Autodesk Inventor part; units mm, degrees
(part 3 of 7)
  line L1708 (-161.6517, 7.6453) -> (-161.371, 7.5772)
  line L1709 (-161.371, 7.5772) -> (-161.0973, 7.4847)
  line L1710 (-161.0973, 7.4847) -> (-160.8323, 7.3684)
  line L1711 (-160.8323, 7.3684) -> (-160.4964, 7.1575)
  line L1712 (-160.4964, 7.1575) -> (-160.1956, 6.9075)
  line L1713 (-160.1956, 6.9075) -> (-159.9378, 6.6106)
  line L1714 (-159.9378, 6.6106) -> (-159.719, 6.2747)
  line L1715 (-159.719, 6.2747) -> (-159.5477, 5.9087)
  line L1716 (-159.5477, 5.9087) -> (-159.4222, 5.5247)
  line L1717 (-159.4222, 5.5247) -> (-159.3479, 5.1262)
  line L1718 (-159.3479, 5.1262) -> (-159.3206, 4.7083)
  line L1719 (-159.3206, 4.7083) -> (-159.3319, 4.394)
  line L1720 (-159.3319, 4.394) -> (-159.3724, 4.0828)
  line L1721 (-159.3724, 4.0828) -> (-159.4417, 3.7767)
  line L1722 (-159.4417, 3.7767) -> (-159.5394, 3.4778)
  line L1723 (-159.5394, 3.4778) -> (-159.6691, 3.2001)
  line L1724 (-159.6691, 3.2001) -> (-159.8274, 2.9409)
  line L1725 (-159.8274, 2.9409) -> (-160.0121, 2.7021)
  line L1726 (-160.0121, 2.7021) -> (-160.2213, 2.4856)
  line L1727 (-160.2213, 2.4856) -> (-160.453, 2.2932)
  line L1728 (-160.453, 2.2932) -> (-160.705, 2.127)
  line L1729 (-160.705, 2.127) -> (-160.9754, 1.9886)
  line L1730 (-160.9754, 1.9886) -> (-161.262, 1.8801)
  line L1731 (-161.262, 1.8801) -> (-161.7812, 1.7492)
  line L1732 (-161.7812, 1.7492) -> (-162.3128, 1.6848)
  line L1733 (-162.3128, 1.6848) -> (-162.7199, 1.6679)
  line L1734 (-162.7199, 1.6679) -> (-163.1263, 1.6832)
  line L1735 (-163.1263, 1.6832) -> (-163.5304, 1.7305)
  line L1736 (-163.5304, 1.7305) -> (-163.93, 1.8098)
  line L1737 (-163.93, 1.8098) -> (-164.1821, 1.8844)
  line L1738 (-164.1821, 1.8844) -> (-164.4265, 1.9799)
  line L1739 (-164.4265, 1.9799) -> (-164.6619, 2.0959)
  line L1740 (-164.6619, 2.0959) -> (-164.887, 2.2317)
  line L1741 (-164.887, 2.2317) -> (-165.1134, 2.4105)
  line L1742 (-165.1134, 2.4105) -> (-165.3189, 2.6097)
  line L1743 (-165.3189, 2.6097) -> (-165.5025, 2.8275)
  line L1744 (-165.5025, 2.8275) -> (-165.6629, 3.062)
  line L1745 (-165.6629, 3.062) -> (-165.7992, 3.3114)
  line L1746 (-165.7992, 3.3114) -> (-165.91, 3.5738)
  line L1747 (-165.91, 3.5738) -> (-165.9944, 3.8473)
  line L1748 (-165.9944, 3.8473) -> (-166.0511, 4.1301)
  line L1749 (-166.0511, 4.1301) -> (-166.0959, 4.5823)
  line L1750 (-166.0959, 4.5823) -> (-166.0823, 5.0364)
  line L1751 (-162.1487, -31.7214) -> (-161.6707, -31.7085)
  line L1752 (-161.6707, -31.7085) -> (-161.1956, -31.655)
  line L1753 (-161.1956, -31.655) -> (-160.9008, -31.547)
  line L1754 (-160.9008, -31.547) -> (-160.6503, -31.367)
  line L1755 (-160.6503, -31.367) -> (-160.4566, -31.1269)
  line L1756 (-160.4566, -31.1269) -> (-160.3323, -30.8386)
  line L1757 (-160.3323, -30.8386) -> (-160.2843, -30.6013)
  line L1758 (-160.2843, -30.6013) -> (-160.2692, -30.363)
  line L1759 (-160.2692, -30.363) -> (-160.2861, -30.1269)
  line L1760 (-160.2861, -30.1269) -> (-160.3342, -29.896)
  line L1761 (-160.3342, -29.896) -> (-160.4126, -29.6737)
  line L1762 (-160.4126, -29.6737) -> (-160.5203, -29.4629)
  line L1763 (-160.5203, -29.4629) -> (-160.6566, -29.2668)
  line L1764 (-160.6566, -29.2668) -> (-160.8206, -29.0886)
  line L1765 (-160.8206, -29.0886) -> (-161.0047, -28.9477)
  line L1766 (-161.0047, -28.9477) -> (-161.2112, -28.8425)
  line L1767 (-161.2112, -28.8425) -> (-161.6426, -28.7268)
  line L1768 (-161.6426, -28.7268) -> (-162.0862, -28.6746)
  line L1769 (-162.0862, -28.6746) -> (-162.4769, -28.6628)
  line L1770 (-162.4769, -28.6628) -> (-165.9495, -28.6628)
  line L1771 (-165.9495, -28.6628) -> (-165.9495, -27.5652)
  line L1772 (-165.9495, -27.5652) -> (-159.469, -27.5652)
  line L1773 (-159.469, -27.5652) -> (-159.469, -28.5496)
  line L1774 (-159.469, -28.5496) -> (-160.4222, -28.5496)
  line L1775 (-160.4222, -28.5496) -> (-160.234, -28.6876)
  line L1776 (-160.234, -28.6876) -> (-160.0587, -28.841)
  line L1777 (-160.0587, -28.841) -> (-159.8971, -29.0088)
  line L1778 (-159.8971, -29.0088) -> (-159.7503, -29.1902)
  line L1779 (-159.7503, -29.1902) -> (-159.5954, -29.4431)
  line L1780 (-159.5954, -29.4431) -> (-159.4745, -29.7126)
  line L1781 (-159.4745, -29.7126) -> (-159.389, -29.9953)
  line L1782 (-159.389, -29.9953) -> (-159.3401, -30.2878)
  line L1783 (-159.3401, -30.2878) -> (-159.3229, -30.7084)
  line L1784 (-159.3229, -30.7084) -> (-159.3716, -31.1238)
  line L1785 (-159.3716, -31.1238) -> (-159.4846, -31.5266)
  line L1786 (-159.4846, -31.5266) -> (-159.6604, -31.9089)
  line L1787 (-159.6604, -31.9089) -> (-159.812, -32.1381)
  line L1788 (-159.812, -32.1381) -> (-159.9997, -32.3358)
  line L1789 (-159.9997, -32.3358) -> (-160.219, -32.4978)
  line L1790 (-160.219, -32.4978) -> (-160.4651, -32.6199)
  line L1791 (-160.4651, -32.6199) -> (-160.7422, -32.7101)
  line L1792 (-160.7422, -32.7101) -> (-161.026, -32.7729)
  line L1793 (-161.026, -32.7729) -> (-161.3145, -32.8081)
  line L1794 (-161.3145, -32.8081) -> (-161.6058, -32.8152)
  line L1795 (-161.6058, -32.8152) -> (-161.9339, -32.8191)
  line L1796 (-161.9339, -32.8191) -> (-165.9495, -32.8191)
  line L1797 (-165.9495, -32.8191) -> (-165.9495, -31.7214)
  line L1798 (-165.9495, -31.7214) -> (-162.1487, -31.7214)
  line L1799 (-166.0823, 18.9309) -> (-166.0294, 19.3048)
  line L1800 (-166.0294, 19.3048) -> (-165.9272, 19.6627)
  line L1801 (-165.9272, 19.6627) -> (-165.7786, 20.0006)
  line L1802 (-165.7786, 20.0006) -> (-165.5867, 20.314)
  line L1803 (-165.5867, 20.314) -> (-165.3544, 20.5989)
  line L1804 (-165.3544, 20.5989) -> (-165.0848, 20.8509)
  line L1805 (-165.0848, 20.8509) -> (-164.7809, 21.0658)
  line L1806 (-164.7809, 21.0658) -> (-164.4456, 21.2395)
  line L1807 (-164.4456, 21.2395) -> (-164.1239, 21.3614)
  line L1808 (-164.1239, 21.3614) -> (-163.7934, 21.4544)
  line L1809 (-163.7934, 21.4544) -> (-163.4559, 21.5181)
  line L1810 (-163.4559, 21.5181) -> (-163.1136, 21.552)
  line L1811 (-163.1136, 21.552) -> (-162.7718, 21.561)
  line L1812 (-162.7718, 21.561) -> (-162.43, 21.5559)
  line L1813 (-162.43, 21.5559) -> (-162.43, 16.7239)
  line L1814 (-162.43, 16.7239) -> (-162.1358, 16.7468)
  line L1815 (-162.1358, 16.7468) -> (-161.8463, 16.7991)
  line L1816 (-161.8463, 16.7991) -> (-161.5634, 16.8801)
  line L1817 (-161.5634, 16.8801) -> (-161.2894, 16.9895)
  line L1818 (-161.2894, 16.9895) -> (-161.0538, 17.1191)
  line L1819 (-161.0538, 17.1191) -> (-160.8431, 17.2792)
  line L1820 (-160.8431, 17.2792) -> (-160.6596, 17.4661)
  line L1821 (-160.6596, 17.4661) -> (-160.5054, 17.6765)
  line L1822 (-160.5054, 17.6765) -> (-160.3829, 17.9067)
  line L1823 (-160.3829, 17.9067) -> (-160.2941, 18.1532)
  line L1824 (-160.2941, 18.1532) -> (-160.2413, 18.4124)
  line L1825 (-160.2413, 18.4124) -> (-160.2269, 18.6809)
  line L1826 (-160.2269, 18.6809) -> (-160.2451, 18.965)
  line L1827 (-160.2451, 18.965) -> (-160.305, 19.2434)
  line L1828 (-160.305, 19.2434) -> (-160.4023, 19.4889)
  line L1829 (-160.4023, 19.4889) -> (-160.5433, 19.7122)
  line L1830 (-160.5433, 19.7122) -> (-160.7325, 19.9205)
  line L1831 (-160.7325, 19.9205) -> (-160.9534, 20.095)
  line L1832 (-160.9534, 20.095) -> (-161.2449, 20.2622)
  line L1833 (-161.2449, 20.2622) -> (-161.555, 20.3918)
  line L1834 (-161.555, 20.3918) -> (-161.4144, 21.5286)
  line L1835 (-161.4144, 21.5286) -> (-161.0762, 21.42)
  line L1836 (-161.0762, 21.42) -> (-160.7548, 21.2719)
  line L1837 (-160.7548, 21.2719) -> (-160.4536, 21.0861)
  line L1838 (-160.4536, 21.0861) -> (-160.1761, 20.8645)
  line L1839 (-160.1761, 20.8645) -> (-159.9008, 20.5641)
  line L1840 (-159.9008, 20.5641) -> (-159.6771, 20.2266)
  line L1841 (-159.6771, 20.2266) -> (-159.5085, 19.8584)
  line L1842 (-159.5085, 19.8584) -> (-159.3987, 19.4661)
  line L1843 (-159.3987, 19.4661) -> (-159.3276, 18.9457)
  line L1844 (-159.3276, 18.9457) -> (-159.3283, 18.4229)
  line L1845 (-159.3283, 18.4229) -> (-159.4004, 17.9051)
  line L1846 (-159.4004, 17.9051) -> (-159.5433, 17.3997)
  line L1847 (-159.5433, 17.3997) -> (-159.6699, 17.1215)
  line L1848 (-159.6699, 17.1215) -> (-159.8254, 16.8617)
  line L1849 (-159.8254, 16.8617) -> (-160.0078, 16.6223)
  line L1850 (-160.0078, 16.6223) -> (-160.215, 16.4051)
  line L1851 (-160.215, 16.4051) -> (-160.4449, 16.2122)
  line L1852 (-160.4449, 16.2122) -> (-160.6955, 16.0454)
  line L1853 (-160.6955, 16.0454) -> (-160.9646, 15.9067)
  line L1854 (-160.9646, 15.9067) -> (-161.2503, 15.7981)
  line L1855 (-161.2503, 15.7981) -> (-161.5947, 15.7031)
  line L1856 (-161.5947, 15.7031) -> (-161.9449, 15.6361)
  line L1857 (-161.9449, 15.6361) -> (-162.2995, 15.5974)
  line L1858 (-162.2995, 15.5974) -> (-162.6565, 15.5872)
  line L1859 (-162.6565, 15.5872) -> (-163.0242, 15.5978)
  line L1860 (-163.0242, 15.5978) -> (-163.3893, 15.6367)
  line L1861 (-163.3893, 15.6367) -> (-163.7504, 15.7035)
  line L1862 (-163.7504, 15.7035) -> (-164.1058, 15.7981)
  line L1863 (-164.1058, 15.7981) -> (-164.3965, 15.9063)
  line L1864 (-164.3965, 15.9063) -> (-164.6712, 16.0443)
  line L1865 (-164.6712, 16.0443) -> (-164.9279, 16.2102)
  line L1866 (-164.9279, 16.2102) -> (-165.1647, 16.4023)
  line L1867 (-165.1647, 16.4023) -> (-165.3794, 16.6187)
  line L1868 (-165.3794, 16.6187) -> (-165.5701, 16.8576)
  line L1869 (-165.5701, 16.8576) -> (-165.7348, 17.1173)
  line L1870 (-165.7348, 17.1173) -> (-165.8714, 17.3958)
  line L1871 (-165.8714, 17.3958) -> (-165.9915, 17.7683)
  line L1872 (-165.9915, 17.7683) -> (-166.0671, 18.1509)
  line L1873 (-166.0671, 18.1509) -> (-166.0976, 18.5398)
  line L1874 (-166.0976, 18.5398) -> (-166.0823, 18.9309)
  line L1875 (-166.0862, -17.1589) -> (-166.0498, -16.8212)
  line L1876 (-166.0498, -16.8212) -> (-165.9886, -16.4871)
  line L1877 (-165.9886, -16.4871) -> (-165.9182, -16.2439)
  line L1878 (-165.9182, -16.2439) -> (-165.8211, -16.011)
  line L1879 (-165.8211, -16.011) -> (-165.6984, -15.7906)
  line L1880 (-165.6984, -15.7906) -> (-165.5511, -15.5847)
  line L1881 (-165.5511, -15.5847) -> (-165.4065, -15.444)
  line L1882 (-165.4065, -15.444) -> (-165.2447, -15.3251)
  line L1883 (-165.2447, -15.3251) -> (-165.0681, -15.2296)
  line L1884 (-165.0681, -15.2296) -> (-164.8792, -15.1589)
  line L1885 (-164.8792, -15.1589) -> (-164.5781, -15.0877)
  line L1886 (-164.5781, -15.0877) -> (-164.2698, -15.0613)
  line L1887 (-164.2698, -15.0613) -> (-163.9594, -15.0488)
  line L1888 (-163.9594, -15.0488) -> (-163.6487, -15.0457)
  line L1889 (-163.6487, -15.0457) -> (-162.4222, -15.0489)
  line L1890 (-162.4222, -15.0489) -> (-161.1956, -15.0378)
  line L1891 (-161.1956, -15.0378) -> (-160.72, -15.0223)
  line L1892 (-160.72, -15.0223) -> (-160.2464, -14.9753)
  line L1893 (-160.2464, -14.9753) -> (-160.0431, -14.933)
  line L1894 (-160.0431, -14.933) -> (-159.845, -14.8724)
  line L1895 (-159.845, -14.8724) -> (-159.6532, -14.7939)
  line L1896 (-159.6532, -14.7939) -> (-159.469, -14.698)
  line L1897 (-159.469, -14.698) -> (-159.469, -15.8464)
  line L1898 (-159.469, -15.8464) -> (-159.6611, -15.9284)
  line L1899 (-159.6611, -15.9284) -> (-159.8595, -15.9923)
  line L1900 (-159.8595, -15.9923) -> (-160.0628, -16.0381)
  line L1901 (-160.0628, -16.0381) -> (-160.2698, -16.0652)
  line L1902 (-160.2698, -16.0652) -> (-159.9385, -16.4923)
  line L1903 (-159.9385, -16.4923) -> (-159.6604, -16.9558)
  line L1904 (-159.6604, -16.9558) -> (-159.5367, -17.2459)
  line L1905 (-159.5367, -17.2459) -> (-159.4406, -17.5441)
  line L1906 (-159.4406, -17.5441) -> (-159.3723, -17.8486)
  line L1907 (-159.3723, -17.8486) -> (-159.332, -18.1574)
  line L1908 (-159.332, -18.1574) -> (-159.3198, -18.4686)
  line L1909 (-159.3198, -18.4686) -> (-159.3358, -18.7803)
  line L1910 (-159.3358, -18.7803) -> (-159.3803, -19.0905)
  line L1911 (-159.3803, -19.0905) -> (-159.4534, -19.3972)
  line L1912 (-159.4534, -19.3972) -> (-159.5274, -19.6029)
  line L1913 (-159.5274, -19.6029) -> (-159.6248, -19.7959)
  line L1914 (-159.6248, -19.7959) -> (-159.7441, -19.9743)
  line L1915 (-159.7441, -19.9743) -> (-159.8836, -20.1365)
  line L1916 (-159.8836, -20.1365) -> (-160.0415, -20.2808)
  line L1917 (-160.0415, -20.2808) -> (-160.2163, -20.4054)
  line L1918 (-160.2163, -20.4054) -> (-160.4063, -20.5085)
  line L1919 (-160.4063, -20.5085) -> (-160.6097, -20.5886)
  line L1920 (-160.6097, -20.5886) -> (-160.9739, -20.6615)
  line L1921 (-160.9739, -20.6615) -> (-161.3419, -20.6623)
  line L1922 (-161.3419, -20.6623) -> (-161.7032, -20.5921)
  line L1923 (-161.7032, -20.5921) -> (-162.0472, -20.4519)
  line L1924 (-162.0472, -20.4519) -> (-162.3151, -20.2729)
  line L1925 (-162.3151, -20.2729) -> (-162.5475, -20.0529)
  line L1926 (-162.5475, -20.0529) -> (-162.7397, -19.7971)
  line L1927 (-162.7397, -19.7971) -> (-162.887, -19.5105)
  line L1928 (-162.887, -19.5105) -> (-162.9874, -19.2476)
  line L1929 (-162.9874, -19.2476) -> (-163.0672, -18.9781)
  line L1930 (-163.0672, -18.9781) -> (-163.1263, -18.7034)
  line L1931 (-163.1263, -18.7034) -> (-163.1644, -18.4246)
  line L1932 (-163.1644, -18.4246) -> (-163.291, -17.4646)
  line L1933 (-163.291, -17.4646) -> (-163.4769, -16.5144)
  line L1934 (-163.4769, -16.5144) -> (-163.5251, -16.3354)
  line L1935 (-163.5251, -16.3354) -> (-163.5823, -16.1589)
  line L1936 (-163.5823, -16.1589) -> (-164.015, -16.158)
  line L1937 (-164.015, -16.158) -> (-164.4417, -16.2293)
  line L1938 (-164.4417, -16.2293) -> (-164.6111, -16.301)
  line L1939 (-164.6111, -16.301) -> (-164.7599, -16.4058)
  line L1940 (-164.7599, -16.4058) -> (-164.8834, -16.5395)
  line L1941 (-164.8834, -16.5395) -> (-164.9769, -16.698)
  line L1942 (-164.9769, -16.698) -> (-165.0615, -16.8928)
  line L1943 (-165.0615, -16.8928) -> (-165.1246, -17.095)
  line L1944 (-165.1246, -17.095) -> (-165.1655, -17.3028)
  line L1945 (-165.1655, -17.3028) -> (-165.1839, -17.5144)
  line L1946 (-165.1839, -17.5144) -> (-165.1827, -17.9541)
  line L1947 (-165.1827, -17.9541) -> (-165.1214, -18.3894)
  line L1948 (-165.1214, -18.3894) -> (-165.0354, -18.6472)
  line L1949 (-165.0354, -18.6472) -> (-164.9183, -18.8582)
  line L1950 (-164.9183, -18.8582) -> (-164.7542, -19.03)
  line L1951 (-164.7542, -19.03) -> (-164.5394, -19.1785)
  line L1952 (-164.5394, -19.1785) -> (-164.2539, -19.3112)
  line L1953 (-164.2539, -19.3112) -> (-163.9534, -19.405)
  line L1954 (-163.9534, -19.405) -> (-164.1019, -20.4793)
  line L1955 (-164.1019, -20.4793) -> (-164.3331, -20.4248)
  line L1956 (-164.3331, -20.4248) -> (-164.5587, -20.3517)
  line L1957 (-164.5587, -20.3517) -> (-164.7776, -20.2603)
  line L1958 (-164.7776, -20.2603) -> (-164.9886, -20.1511)
  line L1959 (-164.9886, -20.1511) -> (-165.1636, -20.0373)
  line L1960 (-165.1636, -20.0373) -> (-165.3233, -19.9039)
  line L1961 (-165.3233, -19.9039) -> (-165.466, -19.7526)
  line L1962 (-165.466, -19.7526) -> (-165.5901, -19.5847)
  line L1963 (-165.5901, -19.5847) -> (-165.7484, -19.3151)
  line L1964 (-165.7484, -19.3151) -> (-165.8675, -19.0261)
  line L1965 (-165.8675, -19.0261) -> (-166.0114, -18.5003)
  line L1966 (-166.0114, -18.5003) -> (-166.0823, -17.9597)
  line L1967 (-166.0823, -17.9597) -> (-166.0979, -17.5594)
  line L1968 (-166.0979, -17.5594) -> (-166.0862, -17.1589)
  line L1969 (-165.9495, -0.1277) -> (-165.9495, 0.9778)
  line L1970 (-165.9495, 0.9778) -> (-165.0979, 0.9778)
  line L1971 (-165.0979, 0.9778) -> (-165.0979, -0.1277)
  line L1972 (-165.0979, -0.1277) -> (-161.305, -0.1277)
  line L1973 (-161.305, -0.1277) -> (-161.0019, -0.1218)
  line L1974 (-161.0019, -0.1218) -> (-160.7034, -0.0691)
  line L1975 (-160.7034, -0.0691) -> (-160.5823, 0.009)
  line L1976 (-160.5823, 0.009) -> (-160.4886, 0.1184)
  line L1977 (-160.4886, 0.1184) -> (-160.4244, 0.3027)
  line L1978 (-160.4244, 0.3027) -> (-160.4104, 0.4973)
  line L1979 (-160.4104, 0.4973) -> (-160.4208, 0.7385)
  line L1980 (-160.4208, 0.7385) -> (-160.4534, 0.9778)
  line L1981 (-160.4534, 0.9778) -> (-159.4808, 1.1379)
  line L1982 (-159.4808, 1.1379) -> (-159.4181, 0.8002)
  line L1983 (-159.4181, 0.8002) -> (-159.3887, 0.4588)
  line L1984 (-159.3887, 0.4588) -> (-159.3926, 0.1161)
  line L1985 (-159.3926, 0.1161) -> (-159.43, -0.2253)
  line L1986 (-159.43, -0.2253) -> (-159.4939, -0.454)
  line L1987 (-159.4939, -0.454) -> (-159.5996, -0.6641)
  line L1988 (-159.5996, -0.6641) -> (-159.7435, -0.8502)
  line L1989 (-159.7435, -0.8502) -> (-159.9222, -1.0066)
  line L1990 (-159.9222, -1.0066) -> (-160.0697, -1.0786)
  line L1991 (-160.0697, -1.0786) -> (-160.2242, -1.1329)
  line L1992 (-160.2242, -1.1329) -> (-160.3838, -1.1689)
  line L1993 (-160.3838, -1.1689) -> (-160.5472, -1.1863)
  line L1994 (-160.5472, -1.1863) -> (-160.8379, -1.2064)
  line L1995 (-160.8379, -1.2064) -> (-161.1292, -1.2175)
  line L1996 (-161.1292, -1.2175) -> (-165.0979, -1.2175)
  line L1997 (-165.0979, -1.2175) -> (-165.0979, -2.0261)
  line L1998 (-165.0979, -2.0261) -> (-165.9495, -2.0261)
  line L1999 (-165.9495, -2.0261) -> (-165.9495, -1.2175)
  line L2000 (-165.9495, -1.2175) -> (-167.555, -1.2175)
  line L2001 (-167.555, -1.2175) -> (-168.2151, -0.1277)
  line L2002 (-168.2151, -0.1277) -> (-165.9495, -0.1277)
  line L2003 (-166.0745, 25.6145) -> (-166.0237, 25.8381)
  line L2004 (-166.0237, 25.8381) -> (-165.951, 26.055)
  line L2005 (-165.951, 26.055) -> (-165.857, 26.2635)
  line L2006 (-165.857, 26.2635) -> (-165.7425, 26.4621)
  line L2007 (-165.7425, 26.4621) -> (-164.7229, 26.0871)
  line L2008 (-164.7229, 26.0871) -> (-164.8424, 25.8584)
  line L2009 (-164.8424, 25.8584) -> (-164.9209, 25.6144)
  line L2010 (-164.9209, 25.6144) -> (-164.957, 25.3607)
  line L2011 (-164.957, 25.3607) -> (-164.9495, 25.1028)
  line L2012 (-164.9495, 25.1028) -> (-164.8482, 24.8038)
  line L2013 (-164.8482, 24.8038) -> (-164.6722, 24.5488)
  line L2014 (-164.6722, 24.5488) -> (-164.4337, 24.3511)
  line L2015 (-164.4337, 24.3511) -> (-164.1448, 24.2239)
  line L2016 (-164.1448, 24.2239) -> (-163.8304, 24.1419)
  line L2017 (-163.8304, 24.1419) -> (-163.5111, 24.0838)
  line L2018 (-163.5111, 24.0838) -> (-163.1884, 24.0499)
  line L2019 (-163.1884, 24.0499) -> (-162.8636, 24.0403)
  line L2020 (-162.8636, 24.0403) -> (-159.469, 24.0403)
  line L2021 (-159.469, 24.0403) -> (-159.469, 22.9426)
  line L2022 (-159.469, 22.9426) -> (-165.9495, 22.9426)
  line L2023 (-165.9495, 22.9426) -> (-165.9495, 23.9309)
  line L2024 (-165.9495, 23.9309) -> (-164.969, 23.9309)
  line L2025 (-164.969, 23.9309) -> (-165.3729, 24.171)
  line L2026 (-165.3729, 24.171) -> (-165.7386, 24.4661)
  line L2027 (-165.7386, 24.4661) -> (-165.8926, 24.6524)
  line L2028 (-165.8926, 24.6524) -> (-166.0057, 24.8634)
  line L2029 (-166.0057, 24.8634) -> (-166.0751, 25.0926)
  line L2030 (-166.0751, 25.0926) -> (-166.0979, 25.3332)
  line L2031 (-166.0979, 25.3332) -> (-166.0745, 25.6145)
  line L2032 (-159.469, -21.9402) -> (-159.469, -23.0418)
  line L2033 (-159.469, -23.0418) -> (-165.9495, -23.0418)
  line L2034 (-165.9495, -23.0418) -> (-165.9495, -21.9402)
  line L2035 (-165.9495, -21.9402) -> (-159.469, -21.9402)
  line L2036 (-159.469, -24.7214) -> (-159.469, -25.8191)
  line L2037 (-159.469, -25.8191) -> (-168.4183, -25.8191)
  line L2038 (-168.4183, -25.8191) -> (-168.4183, -24.7214)
  line L2039 (-168.4183, -24.7214) -> (-159.469, -24.7214)
  line L2040 (-162.6604, -16.3152) -> (-162.4486, -17.1258)
  line L2041 (-162.4486, -17.1258) -> (-162.3089, -17.9519)
  line L2042 (-162.3089, -17.9519) -> (-162.2265, -18.4372)
  line L2043 (-162.2265, -18.4372) -> (-162.0862, -18.9089)
  line L2044 (-162.0862, -18.9089) -> (-161.9426, -19.1525)
  line L2045 (-161.9426, -19.1525) -> (-161.7377, -19.3384)
  line L2046 (-161.7377, -19.3384) -> (-161.4873, -19.456)
  line L2047 (-161.4873, -19.456) -> (-161.2073, -19.4949)
  line L2048 (-161.2073, -19.4949) -> (-161.0015, -19.4764)
  line L2049 (-161.0015, -19.4764) -> (-160.805, -19.4128)
  line L2050 (-160.805, -19.4128) -> (-160.6666, -19.3319)
  line L2051 (-160.6666, -19.3319) -> (-160.5429, -19.2314)
  line L2052 (-160.5429, -19.2314) -> (-160.436, -19.1132)
  line L2053 (-160.436, -19.1132) -> (-160.3479, -18.9793)
  line L2054 (-160.3479, -18.9793) -> (-160.2545, -18.741)
  line L2055 (-160.2545, -18.741) -> (-160.1995, -18.491)
  line L2056 (-160.1995, -18.491) -> (-160.1809, -18.1923)
  line L2057 (-160.1809, -18.1923) -> (-160.1984, -17.8945)
  line L2058 (-160.1984, -17.8945) -> (-160.2516, -17.6011)
  line L2059 (-160.2516, -17.6011) -> (-160.3401, -17.3152)
  line L2060 (-160.3401, -17.3152) -> (-160.4251, -17.1273)
  line L2061 (-160.4251, -17.1273) -> (-160.5289, -16.9499)
  line L2062 (-160.5289, -16.9499) -> (-160.6507, -16.7841)
  line L2063 (-160.6507, -16.7841) -> (-160.7894, -16.6316)
  line L2064 (-160.7894, -16.6316) -> (-160.9931, -16.4671)
  line L2065 (-160.9931, -16.4671) -> (-161.219, -16.3347)
  line L2066 (-161.219, -16.3347) -> (-161.5906, -16.2186)
  line L2067 (-161.5906, -16.2186) -> (-161.9769, -16.1707)
  line L2068 (-161.9769, -16.1707) -> (-162.3498, -16.1584)
  line L2069 (-162.3498, -16.1584) -> (-162.7229, -16.1589)
  line L2070 (-162.7229, -16.1589) -> (-162.6604, -16.3152)
  line L2071 (-165.18, 4.509) -> (-165.1362, 4.2596)
  line L2072 (-165.1362, 4.2596) -> (-165.0591, 4.0222)
  line L2073 (-165.0591, 4.0222) -> (-164.9508, 3.7998)
  line L2074 (-164.9508, 3.7998) -> (-164.8136, 3.5953)
  line L2075 (-164.8136, 3.5953) -> (-164.6496, 3.4115)
  line L2076 (-164.6496, 3.4115) -> (-164.4612, 3.2512)
  line L2077 (-164.4612, 3.2512) -> (-164.2505, 3.1174)
  line L2078 (-164.2505, 3.1174) -> (-164.0198, 3.0129)
  line L2079 (-164.0198, 3.0129) -> (-163.7012, 2.9138)
  line L2080 (-163.7012, 2.9138) -> (-163.3755, 2.8448)
  line L2081 (-163.3755, 2.8448) -> (-163.0448, 2.8061)
  line L2082 (-163.0448, 2.8061) -> (-162.7112, 2.7981)
  line L2083 (-162.7112, 2.7981) -> (-162.4357, 2.8037)
  line L2084 (-162.4357, 2.8037) -> (-162.1615, 2.8284)
  line L2085 (-162.1615, 2.8284) -> (-161.8898, 2.8722)
  line L2086 (-161.8898, 2.8722) -> (-161.6214, 2.9348)
  line L2087 (-161.6214, 2.9348) -> (-161.4121, 3.0059)
  line L2088 (-161.4121, 3.0059) -> (-161.2118, 3.0979)
  line L2089 (-161.2118, 3.0979) -> (-161.0219, 3.2099)
  line L2090 (-161.0219, 3.2099) -> (-160.844, 3.3411)
  line L2091 (-160.844, 3.3411) -> (-160.685, 3.4959)
  line L2092 (-160.685, 3.4959) -> (-160.5479, 3.6672)
  line L2093 (-160.5479, 3.6672) -> (-160.4335, 3.8527)
  line L2094 (-160.4335, 3.8527) -> (-160.3428, 4.05)
  line L2095 (-160.3428, 4.05) -> (-160.2767, 4.2568)
  line L2096 (-160.2767, 4.2568) -> (-160.236, 4.4709)
  line L2097 (-160.236, 4.4709) -> (-160.2217, 4.6898)
  line L2098 (-160.2217, 4.6898) -> (-160.2347, 4.9114)
  line L2099 (-160.2347, 4.9114) -> (-160.3169, 5.2929)
  line L2100 (-160.3169, 5.2929) -> (-160.4795, 5.6426)
  line L2101 (-160.4795, 5.6426) -> (-160.715, 5.9479)
  line L2102 (-160.715, 5.9479) -> (-161.0159, 6.1965)
  line L2103 (-161.0159, 6.1965) -> (-161.218, 6.3163)
  line L2104 (-161.218, 6.3163) -> (-161.4312, 6.4133)
  line L2105 (-161.4312, 6.4133) -> (-161.6535, 6.4869)
  line L2106 (-161.6535, 6.4869) -> (-161.8831, 6.5364)
  line L2107 (-161.8831, 6.5364) -> (-162.3637, 6.6039)
  line L2108 (-162.3637, 6.6039) -> (-162.8474, 6.6166)
  line L2109 (-162.8474, 6.6166) -> (-163.3294, 6.5745)
  line L2110 (-163.3294, 6.5745) -> (-163.805, 6.4778)
  line L2111 (-163.805, 6.4778) -> (-164.1467, 6.3472)
  line L2112 (-164.1467, 6.3472) -> (-164.4558, 6.1573)
  line L2113 (-164.4558, 6.1573) -> (-164.7246, 5.9138)
  line L2114 (-164.7246, 5.9138) -> (-164.9456, 5.6223)
  line L2115 (-164.9456, 5.6223) -> (-165.0704, 5.3607)
  line L2116 (-165.0704, 5.3607) -> (-165.1518, 5.0844)
  line L2117 (-165.1518, 5.0844) -> (-165.1887, 4.7987)
  line L2118 (-165.1887, 4.7987) -> (-165.18, 4.509)
  line L2119 (-165.18, 11.3645) -> (-165.1288, 11.1049)
  line L2120 (-165.1288, 11.1049) -> (-165.0352, 10.8593)
  line L2121 (-165.0352, 10.8593) -> (-164.9017, 10.6329)
  line L2122 (-164.9017, 10.6329) -> (-164.7308, 10.4309)
  line L2123 (-164.7308, 10.4309) -> (-164.4913, 10.2233)
  line L2124 (-164.4913, 10.2233) -> (-164.2237, 10.0572)
  line L2125 (-164.2237, 10.0572) -> (-163.9333, 9.9354)
  line L2126 (-163.9333, 9.9354) -> (-163.6253, 9.8606)
  line L2127 (-163.6253, 9.8606) -> (-163.1496, 9.7976)
  line L2128 (-163.1496, 9.7976) -> (-162.6712, 9.7857)
  line L2129 (-162.6712, 9.7857) -> (-162.1943, 9.825)
  line L2130 (-162.1943, 9.825) -> (-161.7229, 9.9153)
  line L2131 (-161.7229, 9.9153) -> (-161.5179, 9.9765)
  line L2132 (-161.5179, 9.9765) -> (-161.322, 10.0607)
  line L2133 (-161.322, 10.0607) -> (-161.1371, 10.1669)
  line L2134 (-161.1371, 10.1669) -> (-160.9651, 10.2942)
  line L2135 (-160.9651, 10.2942) -> (-160.8151, 10.4359)
  line L2136 (-160.8151, 10.4359) -> (-160.6855, 10.5935)
  line L2137 (-160.6855, 10.5935) -> (-160.5772, 10.7646)
  line L2138 (-160.5772, 10.7646) -> (-160.4912, 10.9472)
  line L2139 (-160.4912, 10.9472) -> (-160.4283, 11.139)
  line L2140 (-160.4283, 11.139) -> (-160.3894, 11.3377)
  line L2141 (-160.3894, 11.3377) -> (-160.3753, 11.5412)
  line L2142 (-160.3753, 11.5412) -> (-160.387, 11.7473)
  line L2143 (-160.387, 11.7473) -> (-160.4305, 11.9818)
  line L2144 (-160.4305, 11.9818) -> (-160.5052, 12.2046)
  line L2145 (-160.5052, 12.2046) -> (-160.6092, 12.413)
  line L2146 (-160.6092, 12.413) -> (-160.7401, 12.6043)
  line L2147 (-160.7401, 12.6043) -> (-160.8961, 12.7759)
  line L2148 (-160.8961, 12.7759) -> (-161.0748, 12.9251)
  line L2149 (-161.0748, 12.9251) -> (-161.2743, 13.0493)
  line L2150 (-161.2743, 13.0493) -> (-161.4925, 13.1458)
  line L2151 (-161.4925, 13.1458) -> (-161.809, 13.239)
  line L2152 (-161.809, 13.239) -> (-162.132, 13.3034)
  line L2153 (-162.132, 13.3034) -> (-162.4594, 13.3389)
  line L2154 (-162.4594, 13.3389) -> (-162.7894, 13.345)
  line L2155 (-162.7894, 13.345) -> (-163.1102, 13.3393)
  line L2156 (-163.1102, 13.3393) -> (-163.4283, 13.3027)
  line L2157 (-163.4283, 13.3027) -> (-163.7414, 13.2355)
  line L2158 (-163.7414, 13.2355) -> (-164.0472, 13.1379)
  line L2159 (-164.0472, 13.1379) -> (-164.3933, 12.9623)
  line L2160 (-164.3933, 12.9623) -> (-164.6908, 12.7197)
  line L2161 (-164.6908, 12.7197) -> (-164.93, 12.4196)
  line L2162 (-164.93, 12.4196) -> (-165.1019, 12.0715)
  line L2163 (-165.1019, 12.0715) -> (-165.1506, 11.8988)
  line L2164 (-165.1506, 11.8988) -> (-165.18, 11.7223)
  line L2165 (-165.18, 11.7223) -> (-165.1899, 11.5437)
  line L2166 (-165.1899, 11.5437) -> (-165.18, 11.3645)
  line L2167 (-165.1878, 18.4426) -> (-165.1434, 18.1758)
  line L2168 (-165.1434, 18.1758) -> (-165.061, 17.9229)
  line L2169 (-165.061, 17.9229) -> (-164.9432, 17.6876)
  line L2170 (-164.9432, 17.6876) -> (-164.793, 17.473)
  line L2171 (-164.793, 17.473) -> (-164.6129, 17.2828)
  line L2172 (-164.6129, 17.2828) -> (-164.4059, 17.1202)
  line L2173 (-164.4059, 17.1202) -> (-164.1747, 16.9888)
  line L2174 (-164.1747, 16.9888) -> (-163.9222, 16.8918)
  line L2175 (-163.9222, 16.8918) -> (-163.6303, 16.8209)
  line L2176 (-163.6303, 16.8209) -> (-163.3323, 16.7825)
  line L2177 (-163.3323, 16.7825) -> (-163.3323, 20.4036)
  line L2178 (-163.3323, 20.4036) -> (-163.6936, 20.3532)
  line L2179 (-163.6936, 20.3532) -> (-164.0472, 20.2629)
  line L2180 (-164.0472, 20.2629) -> (-164.3284, 20.1418)
  line L2181 (-164.3284, 20.1418) -> (-164.5589, 19.9895)
  line L2182 (-164.5589, 19.9895) -> (-164.8336, 19.7111)
  line L2183 (-164.8336, 19.7111) -> (-165.0356, 19.3818)
  line L2184 (-165.0356, 19.3818) -> (-165.1585, 19.0156)
  line L2185 (-165.1585, 19.0156) -> (-165.1956, 18.6262)
  line L2186 (-165.1956, 18.6262) -> (-165.1878, 18.4426)
  line L2187 (-167.1526, -21.9402) -> (-167.1526, -23.0418)
  line L2188 (-167.1526, -23.0418) -> (-168.4183, -23.0418)
  line L2189 (-168.4183, -23.0418) -> (-168.4183, -21.9402)
  line L2190 (-168.4183, -21.9402) -> (-167.1526, -21.9402)
  line L2191 (-167.219, 4.1418) -> (-167.219, 2.9934)
  line L2192 (-167.219, 2.9934) -> (-168.4729, 2.9934)
  line L2193 (-168.4729, 2.9934) -> (-168.4729, 4.1418)
  line L2194 (-168.4729, 4.1418) -> (-167.219, 4.1418)
  line L2195 (-167.219, 6.4192) -> (-167.219, 5.2708)
  line L2196 (-167.219, 5.2708) -> (-168.4729, 5.2708)
  line L2197 (-168.4729, 5.2708) -> (-168.4729, 6.4192)
  line L2198 (-168.4729, 6.4192) -> (-167.219, 6.4192)
  line L2199 (-180.4456, -23.6355) -> (-180.3675, -23.2605)
  line L2200 (-180.3675, -23.2605) -> (-180.2308, -22.905)
  line L2201 (-180.2308, -22.905) -> (-180.0433, -22.5769)
  line L2202 (-180.0433, -22.5769) -> (-179.8089, -22.2761)
  line L2203 (-179.8089, -22.2761) -> (-179.5315, -22.0183)
  line L2204 (-179.5315, -22.0183) -> (-179.2073, -21.7996)
  line L2205 (-179.2073, -21.7996) -> (-178.8401, -21.616)
  line L2206 (-178.8401, -21.616) -> (-178.537, -21.5048)
  line L2207 (-178.537, -21.5048) -> (-178.2267, -21.4174)
  line L2208 (-178.2267, -21.4174) -> (-177.9106, -21.3541)
  line L2209 (-177.9106, -21.3541) -> (-177.5901, -21.3152)
  line L2210 (-177.5901, -21.3152) -> (-177.2384, -21.2939)
  line L2211 (-177.2384, -21.2939) -> (-176.8866, -21.298)
  line L2212 (-176.8866, -21.298) -> (-176.5359, -21.3272)
  line L2213 (-176.5359, -21.3272) -> (-176.1878, -21.3816)
  line L2214 (-176.1878, -21.3816) -> (-175.7586, -21.4935)
  line L2215 (-175.7586, -21.4935) -> (-175.344, -21.6511)
  line L2216 (-175.344, -21.6511) -> (-174.969, -21.8503)
  line L2217 (-174.969, -21.8503) -> (-174.6409, -22.0886)
  line L2218 (-174.6409, -22.0886) -> (-174.3558, -22.3699)
  line L2219 (-174.3558, -22.3699) -> (-174.1214, -22.6863)
  line L2220 (-174.1214, -22.6863) -> (-173.9378, -23.0339)
  line L2221 (-173.9378, -23.0339) -> (-173.805, -23.3855)
  line L2222 (-173.805, -23.3855) -> (-173.7229, -23.7488)
  line L2223 (-173.7229, -23.7488) -> (-173.6956, -24.1199)
  line L2224 (-173.6956, -24.1199) -> (-173.7093, -24.3666)
  line L2225 (-173.7093, -24.3666) -> (-173.7503, -24.6078)
  line L2226 (-173.7503, -24.6078) -> (-173.8178, -24.8414)
  line L2227 (-173.8178, -24.8414) -> (-173.9107, -25.0654)
  line L2228 (-173.9107, -25.0654) -> (-174.0279, -25.2777)
  line L2229 (-174.0279, -25.2777) -> (-174.1686, -25.4761)
  line L2230 (-174.1686, -25.4761) -> (-174.3316, -25.6585)
  line L2231 (-174.3316, -25.6585) -> (-174.5159, -25.823)
  line L2232 (-174.5159, -25.823) -> (-171.3597, -25.823)
  line L2233 (-171.3597, -25.823) -> (-171.3597, -26.9207)
  line L2234 (-171.3597, -26.9207) -> (-180.3245, -26.9207)
  line L2235 (-180.3245, -26.9207) -> (-180.3245, -25.9207)
  line L2236 (-180.3245, -25.9207) -> (-179.4847, -25.9207)
  line L2237 (-179.4847, -25.9207) -> (-179.7014, -25.751)
  line L2238 (-179.7014, -25.751) -> (-179.8984, -25.5598)
  line L2239 (-179.8984, -25.5598) -> (-180.0741, -25.3489)
  line L2240 (-180.0741, -25.3489) -> (-180.2269, -25.1199)
  line L2241 (-180.2269, -25.1199) -> (-180.3122, -24.9355)
  line L2242 (-180.3122, -24.9355) -> (-180.3794, -24.7443)
  line L2243 (-180.3794, -24.7443) -> (-180.4279, -24.5475)
  line L2244 (-180.4279, -24.5475) -> (-180.4573, -24.3464)
  line L2245 (-180.4573, -24.3464) -> (-180.4729, -24.0418)
  line L2246 (-180.4729, -24.0418) -> (-180.4456, -23.6355)
  line L2247 (-180.4456, -30.6355) -> (-180.3675, -30.2605)
  line L2248 (-180.3675, -30.2605) -> (-180.2308, -29.905)
  line L2249 (-180.2308, -29.905) -> (-180.0433, -29.5769)
  line L2250 (-180.0433, -29.5769) -> (-179.8089, -29.2761)
  line L2251 (-179.8089, -29.2761) -> (-179.5315, -29.0183)
  line L2252 (-179.5315, -29.0183) -> (-179.2073, -28.7996)
  line L2253 (-179.2073, -28.7996) -> (-178.8401, -28.616)
  line L2254 (-178.8401, -28.616) -> (-178.537, -28.5048)
  line L2255 (-178.537, -28.5048) -> (-178.2267, -28.4174)
  line L2256 (-178.2267, -28.4174) -> (-177.9106, -28.3541)
  line L2257 (-177.9106, -28.3541) -> (-177.5901, -28.3152)
  line L2258 (-177.5901, -28.3152) -> (-177.2384, -28.2939)
  line L2259 (-177.2384, -28.2939) -> (-176.8866, -28.298)
  line L2260 (-176.8866, -28.298) -> (-176.5359, -28.3272)
  line L2261 (-176.5359, -28.3272) -> (-176.1878, -28.3816)
  line L2262 (-176.1878, -28.3816) -> (-175.7586, -28.4935)
  line L2263 (-175.7586, -28.4935) -> (-175.344, -28.6511)
  line L2264 (-175.344, -28.6511) -> (-174.969, -28.8503)
  line L2265 (-174.969, -28.8503) -> (-174.6409, -29.0886)
  line L2266 (-174.6409, -29.0886) -> (-174.3558, -29.3699)
  line L2267 (-174.3558, -29.3699) -> (-174.1214, -29.6863)
  line L2268 (-174.1214, -29.6863) -> (-173.9378, -30.0339)
  line L2269 (-173.9378, -30.0339) -> (-173.805, -30.3855)
  line L2270 (-173.805, -30.3855) -> (-173.7229, -30.7488)
  line L2271 (-173.7229, -30.7488) -> (-173.6956, -31.1199)
  line L2272 (-173.6956, -31.1199) -> (-173.7093, -31.3666)
  line L2273 (-173.7093, -31.3666) -> (-173.7503, -31.6078)
  line L2274 (-173.7503, -31.6078) -> (-173.8178, -31.8414)
  line L2275 (-173.8178, -31.8414) -> (-173.9107, -32.0654)
  line L2276 (-173.9107, -32.0654) -> (-174.0279, -32.2777)
  line L2277 (-174.0279, -32.2777) -> (-174.1686, -32.4761)
  line L2278 (-174.1686, -32.4761) -> (-174.3316, -32.6585)
  line L2279 (-174.3316, -32.6585) -> (-174.5159, -32.823)
  line L2280 (-174.5159, -32.823) -> (-171.3597, -32.823)
  line L2281 (-171.3597, -32.823) -> (-171.3597, -33.9207)
  line L2282 (-171.3597, -33.9207) -> (-180.3245, -33.9207)
  line L2283 (-180.3245, -33.9207) -> (-180.3245, -32.9207)
  line L2284 (-180.3245, -32.9207) -> (-179.4847, -32.9207)
  line L2285 (-179.4847, -32.9207) -> (-179.7014, -32.751)
  line L2286 (-179.7014, -32.751) -> (-179.8984, -32.5598)
  line L2287 (-179.8984, -32.5598) -> (-180.0741, -32.3489)
  line L2288 (-180.0741, -32.3489) -> (-180.2269, -32.1199)
  line L2289 (-180.2269, -32.1199) -> (-180.3122, -31.9355)
  line L2290 (-180.3122, -31.9355) -> (-180.3794, -31.7443)
  line L2291 (-180.3794, -31.7443) -> (-180.4279, -31.5475)
  line L2292 (-180.4279, -31.5475) -> (-180.4573, -31.3464)
  line L2293 (-180.4573, -31.3464) -> (-180.4729, -31.0418)
  line L2294 (-180.4729, -31.0418) -> (-180.4456, -30.6355)
  line L2295 (-180.4573, 20.6809) -> (-180.4044, 21.0548)
  line L2296 (-180.4044, 21.0548) -> (-180.3022, 21.4127)
  line L2297 (-180.3022, 21.4127) -> (-180.1536, 21.7506)
  line L2298 (-180.1536, 21.7506) -> (-179.9617, 22.064)
  line L2299 (-179.9617, 22.064) -> (-179.7294, 22.3489)
  line L2300 (-179.7294, 22.3489) -> (-179.4598, 22.6009)
  line L2301 (-179.4598, 22.6009) -> (-179.1559, 22.8158)
  line L2302 (-179.1559, 22.8158) -> (-178.8206, 22.9895)
  line L2303 (-178.8206, 22.9895) -> (-178.4989, 23.1114)
  line L2304 (-178.4989, 23.1114) -> (-178.1684, 23.2044)
  line L2305 (-178.1684, 23.2044) -> (-177.8309, 23.2681)
  line L2306 (-177.8309, 23.2681) -> (-177.4886, 23.302)
  line L2307 (-177.4886, 23.302) -> (-177.1468, 23.311)
  line L2308 (-177.1468, 23.311) -> (-176.805, 23.3059)
  line L2309 (-176.805, 23.3059) -> (-176.805, 18.4739)
  line L2310 (-176.805, 18.4739) -> (-176.5108, 18.4968)
  line L2311 (-176.5108, 18.4968) -> (-176.2213, 18.5491)
  line L2312 (-176.2213, 18.5491) -> (-175.9384, 18.6301)
  line L2313 (-175.9384, 18.6301) -> (-175.6644, 18.7395)
  line L2314 (-175.6644, 18.7395) -> (-175.4288, 18.8691)
  line L2315 (-175.4288, 18.8691) -> (-175.2181, 19.0292)
  line L2316 (-175.2181, 19.0292) -> (-175.0346, 19.2161)
  line L2317 (-175.0346, 19.2161) -> (-174.8804, 19.4265)
  line L2318 (-174.8804, 19.4265) -> (-174.7579, 19.6567)
  line L2319 (-174.7579, 19.6567) -> (-174.6691, 19.9032)
  line L2320 (-174.6691, 19.9032) -> (-174.6163, 20.1624)
  line L2321 (-174.6163, 20.1624) -> (-174.6019, 20.4309)
  line L2322 (-174.6019, 20.4309) -> (-174.6201, 20.715)
  line L2323 (-174.6201, 20.715) -> (-174.68, 20.9934)
  line L2324 (-174.68, 20.9934) -> (-174.7773, 21.2389)
  line L2325 (-174.7773, 21.2389) -> (-174.9183, 21.4622)
  line L2326 (-174.9183, 21.4622) -> (-175.1075, 21.6706)
  line L2327 (-175.1075, 21.6706) -> (-175.3284, 21.845)
  line L2328 (-175.3284, 21.845) -> (-175.6199, 22.0122)
  line L2329 (-175.6199, 22.0122) -> (-175.93, 22.1418)
  line L2330 (-175.93, 22.1418) -> (-175.7894, 23.2786)
  line L2331 (-175.7894, 23.2786) -> (-175.4512, 23.17)
  line L2332 (-175.4512, 23.17) -> (-175.1298, 23.0219)
  line L2333 (-175.1298, 23.0219) -> (-174.8286, 22.8361)
  line L2334 (-174.8286, 22.8361) -> (-174.5511, 22.6145)
  line L2335 (-174.5511, 22.6145) -> (-174.2758, 22.3141)
  line L2336 (-174.2758, 22.3141) -> (-174.0521, 21.9766)
  line L2337 (-174.0521, 21.9766) -> (-173.8835, 21.6084)
  line L2338 (-173.8835, 21.6084) -> (-173.7737, 21.2161)
  line L2339 (-173.7737, 21.2161) -> (-173.7026, 20.6957)
  line L2340 (-173.7026, 20.6957) -> (-173.7033, 20.1729)
  line L2341 (-173.7033, 20.1729) -> (-173.7754, 19.6551)
  line L2342 (-173.7754, 19.6551) -> (-173.9183, 19.1497)
  line L2343 (-173.9183, 19.1497) -> (-174.0449, 18.8715)
  line L2344 (-174.0449, 18.8715) -> (-174.2004, 18.6117)
  line L2345 (-174.2004, 18.6117) -> (-174.3828, 18.3723)
  line L2346 (-174.3828, 18.3723) -> (-174.59, 18.1551)
  line L2347 (-174.59, 18.1551) -> (-174.8199, 17.9622)
  line L2348 (-174.8199, 17.9622) -> (-175.0705, 17.7954)
  line L2349 (-175.0705, 17.7954) -> (-175.3396, 17.6567)
  line L2350 (-175.3396, 17.6567) -> (-175.6253, 17.5481)
  line L2351 (-175.6253, 17.5481) -> (-175.9697, 17.4531)
  line L2352 (-175.9697, 17.4531) -> (-176.3199, 17.3861)
  line L2353 (-176.3199, 17.3861) -> (-176.6745, 17.3474)
  line L2354 (-176.6745, 17.3474) -> (-177.0315, 17.3372)
  line L2355 (-177.0315, 17.3372) -> (-177.3992, 17.3478)
  line L2356 (-177.3992, 17.3478) -> (-177.7643, 17.3867)
  line L2357 (-177.7643, 17.3867) -> (-178.1254, 17.4535)
  line L2358 (-178.1254, 17.4535) -> (-178.4808, 17.5481)
  line L2359 (-178.4808, 17.5481) -> (-178.7715, 17.6563)
  line L2360 (-178.7715, 17.6563) -> (-179.0462, 17.7943)
  line L2361 (-179.0462, 17.7943) -> (-179.3029, 17.9602)
  line L2362 (-179.3029, 17.9602) -> (-179.5397, 18.1523)
  line L2363 (-179.5397, 18.1523) -> (-179.7544, 18.3687)
  line L2364 (-179.7544, 18.3687) -> (-179.9451, 18.6076)
  line L2365 (-179.9451, 18.6076) -> (-180.1098, 18.8673)
  line L2366 (-180.1098, 18.8673) -> (-180.2464, 19.1458)
  line L2367 (-180.2464, 19.1458) -> (-180.3665, 19.5183)
  line L2368 (-180.3665, 19.5183) -> (-180.4421, 19.9009)
  line L2369 (-180.4421, 19.9009) -> (-180.4726, 20.2898)
  line L2370 (-180.4726, 20.2898) -> (-180.4573, 20.6809)
  line L2371 (-180.4573, 37.4309) -> (-180.4044, 37.8048)
  line L2372 (-180.4044, 37.8048) -> (-180.3022, 38.1627)
  line L2373 (-180.3022, 38.1627) -> (-180.1536, 38.5006)
  line L2374 (-180.1536, 38.5006) -> (-179.9617, 38.814)
  line L2375 (-179.9617, 38.814) -> (-179.7294, 39.0989)
  line L2376 (-179.7294, 39.0989) -> (-179.4598, 39.3509)
  line L2377 (-179.4598, 39.3509) -> (-179.1559, 39.5658)
  line L2378 (-179.1559, 39.5658) -> (-178.8206, 39.7395)
  line L2379 (-178.8206, 39.7395) -> (-178.4989, 39.8614)
  line L2380 (-178.4989, 39.8614) -> (-178.1684, 39.9544)
  line L2381 (-178.1684, 39.9544) -> (-177.8309, 40.0181)
  line L2382 (-177.8309, 40.0181) -> (-177.4886, 40.052)
  line L2383 (-177.4886, 40.052) -> (-177.1468, 40.061)
  line L2384 (-177.1468, 40.061) -> (-176.805, 40.0559)
  line L2385 (-176.805, 40.0559) -> (-176.805, 35.2239)
  line L2386 (-176.805, 35.2239) -> (-176.5108, 35.2468)
  line L2387 (-176.5108, 35.2468) -> (-176.2213, 35.2991)
  line L2388 (-176.2213, 35.2991) -> (-175.9384, 35.3801)
  line L2389 (-175.9384, 35.3801) -> (-175.6644, 35.4895)
  line L2390 (-175.6644, 35.4895) -> (-175.4288, 35.6191)
  line L2391 (-175.4288, 35.6191) -> (-175.2181, 35.7792)
  line L2392 (-175.2181, 35.7792) -> (-175.0346, 35.9661)
  line L2393 (-175.0346, 35.9661) -> (-174.8804, 36.1765)
  line L2394 (-174.8804, 36.1765) -> (-174.7579, 36.4067)
  line L2395 (-174.7579, 36.4067) -> (-174.6691, 36.6532)
  line L2396 (-174.6691, 36.6532) -> (-174.6163, 36.9124)
  line L2397 (-174.6163, 36.9124) -> (-174.6019, 37.1809)
  line L2398 (-174.6019, 37.1809) -> (-174.6201, 37.465)
  line L2399 (-174.6201, 37.465) -> (-174.68, 37.7434)
  line L2400 (-174.68, 37.7434) -> (-174.7773, 37.9889)
  line L2401 (-174.7773, 37.9889) -> (-174.9183, 38.2121)
  line L2402 (-174.9183, 38.2121) -> (-175.1075, 38.4206)
  line L2403 (-175.1075, 38.4206) -> (-175.3284, 38.595)
  line L2404 (-175.3284, 38.595) -> (-175.6199, 38.7622)
  line L2405 (-175.6199, 38.7622) -> (-175.93, 38.8918)
  line L2406 (-175.93, 38.8918) -> (-175.7894, 40.0286)
  line L2407 (-175.7894, 40.0286) -> (-175.4512, 39.92)
  line L2408 (-175.4512, 39.92) -> (-175.1298, 39.7719)
  line L2409 (-175.1298, 39.7719) -> (-174.8286, 39.5861)
  line L2410 (-174.8286, 39.5861) -> (-174.5511, 39.3645)
  line L2411 (-174.5511, 39.3645) -> (-174.2758, 39.0641)
  line L2412 (-174.2758, 39.0641) -> (-174.0521, 38.7266)
  line L2413 (-174.0521, 38.7266) -> (-173.8835, 38.3584)
  line L2414 (-173.8835, 38.3584) -> (-173.7737, 37.9661)
  line L2415 (-173.7737, 37.9661) -> (-173.7026, 37.4457)
  line L2416 (-173.7026, 37.4457) -> (-173.7033, 36.9229)
  line L2417 (-173.7033, 36.9229) -> (-173.7754, 36.4051)
  line L2418 (-173.7754, 36.4051) -> (-173.9183, 35.8996)
  line L2419 (-173.9183, 35.8996) -> (-174.0449, 35.6215)
  line L2420 (-174.0449, 35.6215) -> (-174.2004, 35.3617)
  line L2421 (-174.2004, 35.3617) -> (-174.3828, 35.1223)
  line L2422 (-174.3828, 35.1223) -> (-174.59, 34.9051)
  line L2423 (-174.59, 34.9051) -> (-174.8199, 34.7122)
  line L2424 (-174.8199, 34.7122) -> (-175.0705, 34.5454)
  line L2425 (-175.0705, 34.5454) -> (-175.3396, 34.4067)
  line L2426 (-175.3396, 34.4067) -> (-175.6253, 34.2981)
  line L2427 (-175.6253, 34.2981) -> (-175.9697, 34.2031)
  line L2428 (-175.9697, 34.2031) -> (-176.3199, 34.1361)
  line L2429 (-176.3199, 34.1361) -> (-176.6745, 34.0974)
  line L2430 (-176.6745, 34.0974) -> (-177.0315, 34.0871)
  line L2431 (-177.0315, 34.0871) -> (-177.3992, 34.0978)
  line L2432 (-177.3992, 34.0978) -> (-177.7643, 34.1367)
  line L2433 (-177.7643, 34.1367) -> (-178.1254, 34.2035)
  line L2434 (-178.1254, 34.2035) -> (-178.4808, 34.2981)
  line L2435 (-178.4808, 34.2981) -> (-178.7715, 34.4063)
  line L2436 (-178.7715, 34.4063) -> (-179.0462, 34.5443)
  line L2437 (-179.0462, 34.5443) -> (-179.3029, 34.7102)
  line L2438 (-179.3029, 34.7102) -> (-179.5397, 34.9023)
  line L2439 (-179.5397, 34.9023) -> (-179.7544, 35.1187)
  line L2440 (-179.7544, 35.1187) -> (-179.9451, 35.3576)
  line L2441 (-179.9451, 35.3576) -> (-180.1098, 35.6173)
  line L2442 (-180.1098, 35.6173) -> (-180.2464, 35.8957)
  line L2443 (-180.2464, 35.8957) -> (-180.3665, 36.2683)
  line L2444 (-180.3665, 36.2683) -> (-180.4421, 36.6509)
  line L2445 (-180.4421, 36.6509) -> (-180.4726, 37.0398)
  line L2446 (-180.4726, 37.0398) -> (-180.4573, 37.4309)
  line L2447 (-180.4573, 10.4543) -> (-180.4231, 10.7749)
  line L2448 (-180.4231, 10.7749) -> (-180.3573, 11.0897)
  line L2449 (-180.3573, 11.0897) -> (-180.2604, 11.3964)
  line L2450 (-180.2604, 11.3964) -> (-180.1331, 11.6926)
  line L2451 (-180.1331, 11.6926) -> (-180, 11.9162)
  line L2452 (-180, 11.9162) -> (-179.8362, 12.1184)
  line L2453 (-179.8362, 12.1184) -> (-179.6987, 12.241)
  line L2454 (-179.6987, 12.241) -> (-179.5491, 12.3476)
  line L2455 (-179.5491, 12.3476) -> (-179.3887, 12.4372)
  line L2456 (-179.3887, 12.4372) -> (-179.219, 12.509)
  line L2457 (-179.219, 12.509) -> (-178.9393, 12.5947)
  line L2458 (-178.9393, 12.5947) -> (-178.6526, 12.6536)
  line L2459 (-178.6526, 12.6536) -> (-178.5081, 11.5793)
  line L2460 (-178.5081, 11.5793) -> (-178.7363, 11.5266)
  line L2461 (-178.7363, 11.5266) -> (-178.9534, 11.4387)
  line L2462 (-178.9534, 11.4387) -> (-179.0938, 11.3467)
  line L2463 (-179.0938, 11.3467) -> (-179.2181, 11.2352)
  line L2464 (-179.2181, 11.2352) -> (-179.3243, 11.1063)
  line L2465 (-179.3243, 11.1063) -> (-179.4104, 10.9622)
  line L2466 (-179.4104, 10.9622) -> (-179.5003, 10.7317)
  line L2467 (-179.5003, 10.7317) -> (-179.5572, 10.3965)
  line L2468 (-179.5572, 10.3965) -> (-179.5715, 10.0581)
  line L2469 (-179.5715, 10.0581) -> (-179.5434, 9.7206)
  line L2470 (-179.5434, 9.7206) -> (-179.4729, 9.3879)
  line L2471 (-179.4729, 9.3879) -> (-179.3887, 9.1851)
  line L2472 (-179.3887, 9.1851) -> (-179.2598, 9.0112)
  line L2473 (-179.2598, 9.0112) -> (-179.0929, 8.8734)
  line L2474 (-179.0929, 8.8734) -> (-178.8948, 8.7786)
  line L2475 (-178.8948, 8.7786) -> (-178.69, 8.7629)
  line L2476 (-178.69, 8.7629) -> (-178.4949, 8.8095)
  line L2477 (-178.4949, 8.8095) -> (-178.3229, 8.913)
  line L2478 (-178.3229, 8.913) -> (-178.1878, 9.0676)
  line L2479 (-178.1878, 9.0676) -> (-178.047, 9.3451)
  line L2480 (-178.047, 9.3451) -> (-177.9534, 9.6418)
  line L2481 (-177.9534, 9.6418) -> (-177.6773, 10.6442)
  line L2482 (-177.6773, 10.6442) -> (-177.3714, 11.6379)
  line L2483 (-177.3714, 11.6379) -> (-177.2871, 11.8746)
  line L2484 (-177.2871, 11.8746) -> (-177.1739, 12.0978)
  line L2485 (-177.1739, 12.0978) -> (-177.0335, 12.305)
  line L2486 (-177.0335, 12.305) -> (-176.8675, 12.4934)
  line L2487 (-176.8675, 12.4934) -> (-176.6809, 12.6421)
  line L2488 (-176.6809, 12.6421) -> (-176.4738, 12.7574)
  line L2489 (-176.4738, 12.7574) -> (-176.2507, 12.8374)
  line L2490 (-176.2507, 12.8374) -> (-176.0159, 12.8801)
  line L2491 (-176.0159, 12.8801) -> (-175.7453, 12.8984)
  line L2492 (-175.7453, 12.8984) -> (-175.4763, 12.8767)
  line L2493 (-175.4763, 12.8767) -> (-175.2135, 12.8157)
  line L2494 (-175.2135, 12.8157) -> (-174.9612, 12.7161)
  line L2495 (-174.9612, 12.7161) -> (-174.7693, 12.6131)
  line L2496 (-174.7693, 12.6131) -> (-174.591, 12.4893)
  line L2497 (-174.591, 12.4893) -> (-174.4278, 12.3462)
  line L2498 (-174.4278, 12.3462) -> (-174.2815, 12.1848)
  line L2499 (-174.2815, 12.1848) -> (-174.1426, 11.9905)
  line L2500 (-174.1426, 11.9905) -> (-174.0235, 11.7842)
  line L2501 (-174.0235, 11.7842) -> (-173.925, 11.5672)
  line L2502 (-173.925, 11.5672) -> (-173.8479, 11.3411)
  line L2503 (-173.8479, 11.3411) -> (-173.7661, 11.0061)
  line L2504 (-173.7661, 11.0061) -> (-173.7152, 10.6659)
  line L2505 (-173.7152, 10.6659) -> (-173.6955, 10.3224)
  line L2506 (-173.6955, 10.3224) -> (-173.7073, 9.9778)
  line L2507 (-173.7073, 9.9778) -> (-173.7309, 9.6557)
  line L2508 (-173.7309, 9.6557) -> (-173.7867, 9.3384)
  line L2509 (-173.7867, 9.3384) -> (-173.8741, 9.0283)
  line L2510 (-173.8741, 9.0283) -> (-173.9925, 8.7278)
  line L2511 (-173.9925, 8.7278) -> (-174.191, 8.4041)
  line L2512 (-174.191, 8.4041) -> (-174.4428, 8.124)
  line L2513 (-174.4428, 8.124) -> (-174.7409, 7.8939)
  line L2514 (-174.7409, 7.8939) -> (-175.0784, 7.72)
  line L2515 (-175.0784, 7.72) -> (-175.4222, 7.5969)
  line L2516 (-175.4222, 7.5969) -> (-175.7776, 7.5129)
  line L2517 (-175.7776, 7.5129) -> (-175.9495, 8.6028)
  line L2518 (-175.9495, 8.6028) -> (-175.6409, 8.6692)
  line L2519 (-175.6409, 8.6692) -> (-175.3714, 8.7747)
  line L2520 (-175.3714, 8.7747) -> (-175.1409, 8.9231)
  line L2521 (-175.1409, 8.9231) -> (-174.9495, 9.1106)
  line L2522 (-174.9495, 9.1106) -> (-174.7972, 9.3411)
  line L2523 (-174.7972, 9.3411) -> (-174.6878, 9.6106)
  line L2524 (-174.6878, 9.6106) -> (-174.6214, 9.9231)
  line L2525 (-174.6214, 9.9231) -> (-174.6015, 10.1781)
  line L2526 (-174.6015, 10.1781) -> (-174.604, 10.4333)
  line L2527 (-174.604, 10.4333) -> (-174.6289, 10.6874)
  line L2528 (-174.6289, 10.6874) -> (-174.6761, 10.9387)
  line L2529 (-174.6761, 10.9387) -> (-174.7737, 11.1965)
  line L2530 (-174.7737, 11.1965) -> (-174.9104, 11.4036)
  line L2531 (-174.9104, 11.4036) -> (-175.0626, 11.5572)
  line L2532 (-175.0626, 11.5572) -> (-175.2425, 11.677)
  line L2533 (-175.2425, 11.677) -> (-175.43, 11.7473)
  line L2534 (-175.43, 11.7473) -> (-175.6331, 11.7708)
  line L2535 (-175.6331, 11.7708) -> (-175.8038, 11.7486)
  line L2536 (-175.8038, 11.7486) -> (-175.9651, 11.6887)
  line L2537 (-175.9651, 11.6887) -> (-176.0933, 11.5897)
  line L2538 (-176.0933, 11.5897) -> (-176.2002, 11.4699)
  line L2539 (-176.2002, 11.4699) -> (-176.2832, 11.3325)
  line L2540 (-176.2832, 11.3325) -> (-176.3401, 11.1809)
  line L2541 (-176.3401, 11.1809) -> (-176.552, 10.4755)
  line L2542 (-176.552, 10.4755) -> (-176.7386, 9.7629)
  line L2543 (-176.7386, 9.7629) -> (-176.9083, 9.1977)
  line L2544 (-176.9083, 9.1977) -> (-177.1175, 8.6458)
  line L2545 (-177.1175, 8.6458) -> (-177.201, 8.4862)
  line L2546 (-177.201, 8.4862) -> (-177.3011, 8.3371)
  line L2547 (-177.3011, 8.3371) -> (-177.4168, 8.1997)
  line L2548 (-177.4168, 8.1997) -> (-177.5472, 8.0754)
  line L2549 (-177.5472, 8.0754) -> (-177.7774, 7.9169)
  line L2550 (-177.7774, 7.9169) -> (-178.0253, 7.8008)
  line L2551 (-178.0253, 7.8008) -> (-178.2856, 7.7273)
  line L2552 (-178.2856, 7.7273) -> (-178.5529, 7.6966)
  line L2553 (-178.5529, 7.6966) -> (-178.8216, 7.7088)
  line L2554 (-178.8216, 7.7088) -> (-179.0863, 7.7642)
  line L2555 (-179.0863, 7.7642) -> (-179.3418, 7.8629)
  line L2556 (-179.3418, 7.8629) -> (-179.5823, 8.0051)
  line L2557 (-179.5823, 8.0051) -> (-179.8091, 8.1917)
  line L2558 (-179.8091, 8.1917) -> (-180.0022, 8.4105)
  line L2559 (-180.0022, 8.4105) -> (-180.1582, 8.6571)
  line L2560 (-180.1582, 8.6571) -> (-180.2737, 8.927)
  line L2561 (-180.2737, 8.927) -> (-180.3824, 9.2995)
  line L2562 (-180.3824, 9.2995) -> (-180.4495, 9.6806)
  line L2563 (-180.4495, 9.6806) -> (-180.4746, 10.0667)
  line L2564 (-180.4746, 10.0667) -> (-180.4573, 10.4543)
  line L2565 (-180.3245, 15.4973) -> (-180.3245, 16.6028)
  line L2566 (-180.3245, 16.6028) -> (-179.4729, 16.6028)
  line L2567 (-179.4729, 16.6028) -> (-179.4729, 15.4973)
  line L2568 (-179.4729, 15.4973) -> (-175.68, 15.4973)
  line L2569 (-175.68, 15.4973) -> (-175.3769, 15.5032)
  line L2570 (-175.3769, 15.5032) -> (-175.0784, 15.5559)